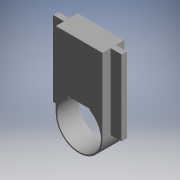
# Autodesk Inventor part: Ajuste
Saved by Autodesk Inventor 2019.3 (Build 233278000, 278)
## iProperties
Part Number: Ajuste
Material: Generic
Document SubType Name: Modeling
Designer: Usuario
Appearance: Default
Author: Usuario
Autodesk Inventor part; units mm, degrees
ref_plane "YZ Plane" through (0, 0, 0) normal (1, 0, 0) x (0, 1, 0)
ref_plane "XZ Plane" through (0, 0, 0) normal (0, 1, 0) x (-1, 0, 0)
ref_plane "XY Plane" through (0, 0, 0) normal (0, 0, 1) x (1, 0, 0)
sketch "Sketch1" plane through (0, 0, 0) normal (0, 0, 1) x (1, 0, 0)
  arc A0 (-12.7, 21.997) -> (12.7, 21.997) centre (0, 0) ccw
  arc A1 (-26.9875, 0) -> (26.9875, 0) centre (0, 0) ccw
  line L0 (-12.7, 23.8125) -> (12.7, 23.8125)
  line L1 (-26.9875, 0) -> (-26.9875, 87.376)
  line L2 (26.9875, 0) -> (26.9875, 87.376)
  line L3 (-26.9875, 87.376) -> (26.9875, 87.376)
  line L4 (-12.7, 21.997) -> (-12.7, 23.8125)
  line L5 (12.7, 21.997) -> (12.7, 23.8125)
  point P0 (0, 16.2052)
  dimension "d0" = 53.975
  dimension "d1" = 87.376
  constraints: 12 end point, 4 point on circle, 2 centre point, 2 coincident, 2 vertical, 1 horizontal, 1 parallel, 1 perpendicular, 1 tangent
  measures "d0" diameter of A1
  measures "d1" distance of L1.start L1.end
extrude "Extrusion1" add sketch "Sketch1" along normal blind 25.4
sketch "Sketch2" plane through (-26.9875, 87.376, 0) normal (0, 1, 0) x (1, 0, 0)
  line L0 (53.975, 0) -> (0, 0) projected
  line L1 (0, 0) -> (0, -25.4) projected
  line L2 (0, -9.525) -> (0, -15.875)
  line L3 (0, -12.7) -> (-12.7, -12.7) construction
  line L4 (0, -15.875) -> (-12.7, -15.875)
  line L5 (-12.7, -15.875) -> (-12.7, -9.525)
  line L6 (-12.7, -9.525) -> (0, -9.525)
  line L7 (26.9875, 0) -> (26.9875, -25.4)
  line L8 (53.975, -9.525) -> (53.975, -15.875)
  line L9 (53.975, -9.525) -> (53.975, -15.875)
  line L10 (53.975, -12.7) -> (66.675, -12.7) construction
  line L11 (53.975, -15.875) -> (66.675, -15.875)
  line L12 (66.675, -15.875) -> (66.675, -9.525)
  line L13 (66.675, -9.525) -> (53.975, -9.525)
  point P0 (53.975, -25.4)
  point P1 (53.975, -25.4)
  dimension "d5" = 12.7
  constraints: 24 end point, 7 symmetric about line, 3 perpendicular, 2 midpoint, 1 horizontal, 1 vertical
  measures "d5" distance of L3.start L3.end
extrude "Extrusion3" add sketch "Sketch2" against normal blind 87.376
body "Solid1"
